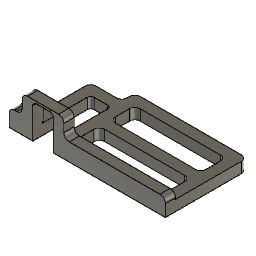
model (Autodesk Fusion 360 design; units mm, degrees)
Autodesk Fusion 360 part; units mm, degrees
note: some values were not read from the file. Set by a fixed rule: which sketch regions a step uses.
sketch "Sketch2" plane through (0, 0, 0) normal (0, 0, 1) x (1, 0, 0) in component "jig"
  line L0 (0, 0) -> (0, 66.75)
  line L1 (0, 66.75) -> (146.025, 66.75)
  line L2 (146.025, 66.75) -> (146.025, 0)
  line L3 (146.025, 0) -> (0, 0)
  line L4 (22.25, 0) -> (41.25, 0)
  line L5 (41.25, 0) -> (41.25, 44.5)
  line L6 (41.25, 44.5) -> (22.25, 44.5)
  line L7 (22.25, 44.5) -> (22.25, 0)
  line L8 (0, 0) -> (22.25, 0)
  line L9 (22.25, 0) -> (22.25, -9.5)
  line L10 (22.25, -9.5) -> (0, -9.5)
  line L11 (0, -9.5) -> (0, 0)
  line L12 (146.025, 0) -> (41.25, 0)
  line L13 (41.25, 0) -> (41.25, -9.5)
  line L14 (41.25, -9.5) -> (146.025, -9.5)
  line L15 (146.025, -9.5) -> (146.025, 0)
  line L16 (22.25, 44.5) -> (0, 44.5) construction
  line L17 (41.25, 44.5) -> (146.025, 44.5) construction
  dimension "d27" = 104.775
  dimension "d29" = 9.5
  dimension "d58" = 19
  dimension "d59" = 22.25
  dimension "d60" = 44.5
  dimension "d64" = 22.25
  constraint coincident L0.start L3.end
  constraint vertical L0
  constraint perpendicular L0 L1
  constraint perpendicular L1 L2
  constraint perpendicular L0 L3
  constraint horizontal L4
  constraint vertical L5
  constraint horizontal L6
  constraint vertical L7
  constraint coincident L3 L4.start
  constraint horizontal L8
  constraint vertical L9
  constraint horizontal L10
  constraint vertical L11
  constraint horizontal L12
  constraint vertical L13
  constraint horizontal L14
  constraint vertical L15
  constraint collinear L10 L14
  constraint collinear L7 L9
  constraint collinear L5 L13
  constraint perpendicular L0 L16
  constraint coincident L0 L16.end
  constraint coincident L2 L17.end
  constraint perpendicular L2 L17
  measures "d27" distance of L2 L5
  measures "d29" distance of L0.start L10.end
  measures "d58" distance of L5.end L6.end
  measures "d59" distance of L1 L6
  measures "d60" distance of L3 L6
  measures "d64" distance of L9.end L10.end
extrude "Extrude1" add sketch "Sketch2" along normal blind 10 contours L0 L1 L2 L3 L5 L6 L7 L8 L12 in component "jig"
extrude "Extrude2" add sketch "Sketch2" along normal blind 33.75 contours L3 L8 L9 L10 L11 | L3 L12 L13 L14 L15 in component "jig"
sketch "Sketch3" plane through (0, 0, 0) normal (-1, 0, 0) x (0, -1, 0) in component "jig"
  line L0 (-66.75, 0) -> (9.5, 0)
  line L1 (9.5, 0) -> (9.5, 33.75)
  line L2 (9.5, 33.75) -> (0, 33.75)
  line L3 (-160, 13) -> (-160.4879, 12.5121)
  line L4 (-160.2757, 12) -> (-160, 12)
  line L5 (-160, 13) -> (-160, 12)
  arc A0 (-160.4879, 12.5121) -> (-160.2757, 12) centre (-160.2757, 12.3) ccw
  line L6 (0, 10) -> (0.2757, 10)
  line L7 (0.4879, 10.5121) -> (0, 11)
  line L8 (0, 10) -> (0, 11)
  arc A1 (0.2757, 10) -> (0.4879, 10.5121) centre (0.2757, 10.3) ccw
  line L9 (-66.75, 10) -> (-66.75, 0)
  line L10 (0, 33.75) -> (0, 10)
  line L11 (0, 10) -> (-66.75, 10)
  dimension "d34" = 1
  dimension "d35" = 0.3
  dimension "d36" = 45
  dimension "d37" = 1
  dimension "d38" = 45
  dimension "d39" = 0.3
  constraint tangent L3 A0
  constraint tangent L4 A0
  constraint tangent L6 A1
  constraint tangent L7 A1
  constraint coincident L6.start L8.start
  measures "d34" distance of L3.start L4.end
  measures "d35" radius of A0
  measures "d36" angle of L3 L5
  measures "d37" distance of L6.start L7.end
  measures "d38" angle of L7 L8
  measures "d39" radius of A1
  measures "d86" radius of A0.centre
extrude "Extrude3" cut sketch "Sketch3" against normal up to surface (146.025 mm away) contours L6 L7 L8 A1 L10 | L3 L4 L5 A0 in component "jig"
fillet "Fillet2" radius 3.175 2 edges at (22.25, 44.5, 5) (41.25, 44.5, 5) in component "jig"
sketch "Sketch2 (2)" plane through (0, -9.5, 0) normal (0, -1, 0) x (1, 0, 0) in component "jig"
  line L0 (0, 0) -> (22.25, 0)
  line L1 (22.25, 0) -> (22.25, 33.75)
  line L2 (22.25, 33.75) -> (0, 33.75)
  line L3 (0, 33.75) -> (0, 0)
  line L4 (22.25, 33.75) -> (41.25, 33.75)
  line L5 (41.25, 0) -> (41.25, 33.75)
  line L6 (41.25, 33.75) -> (41.25, 29.75)
  line L7 (22.25, 33.75) -> (22.25, 29.75)
  line L8 (22.25, 29.75) -> (24.6335, 31.75)
  line L9 (24.6335, 31.75) -> (38.8665, 31.75)
  line L10 (38.8665, 31.75) -> (41.25, 29.75)
  line L11 (22.25, 29.75) -> (41.25, 29.75) construction
  point P0 (41.25, 33.75)
  dimension "d65" = 50
  dimension "d66" = 50
  dimension "d67" = 4
  dimension "d68" = 2
  constraint coincident L1.end L2.start
  constraint coincident P0 L4.end
  constraint coincident L5 L6.end
  constraint perpendicular L4 L6
  constraint coincident L1 L7.end
  constraint perpendicular L2 L7
  constraint perpendicular L1 L9
  constraint horizontal L11
  measures "d65" angle of L7 L8
  measures "d66" angle of L6 L10
  measures "d67" distance of L1.end L7.end
  measures "d68" distance of L4 L9
extrude "Extrude5" add sketch "Sketch2 (2)" against normal up to surface (9.5 mm away) contours L1 L4 L5 L6 L7 L8 L9 L10 in component "jig"
sketch "Sketch3 (2)" plane through (0, 0, 10) normal (0, 0, 1) x (-1, 0, 0) in component "jig"
  line L0 (-25.425, -44.5) -> (-38.075, -44.5)
  arc A0 (-41.25, -41.325) -> (-38.075, -44.5) centre (-38.075, -41.325) ccw
  line L1 (-41.25, -41.325) -> (-41.25, 0.2757)
  line L2 (-41.25, 0.2757) -> (-146.025, 0.2757)
  line L3 (-146.025, 0.2757) -> (-146.025, -66.75)
  line L4 (-146.025, -66.75) -> (0, -66.75)
  line L5 (0, -66.75) -> (0, 0.2757)
  line L6 (0, 0.2757) -> (-22.25, 0.2757)
  line L7 (-22.25, 0.2757) -> (-22.25, -41.325)
  arc A1 (-25.425, -44.5) -> (-22.25, -41.325) centre (-25.425, -41.325) ccw
  line L8 (-56.25, -56.75) -> (-131.025, -56.75)
  line L9 (-136.025, -51.75) -> (-136.025, -38.625)
  line L10 (-131.025, -33.625) -> (-56.25, -33.625)
  line L11 (-51.25, -38.625) -> (-51.25, -51.75)
  line L12 (-146.025, 0) -> (0, 0)
  arc A2 (-56.25, -56.75) -> (-51.25, -51.75) centre (-56.25, -51.75) ccw
  arc A3 (-136.025, -51.75) -> (-131.025, -56.75) centre (-131.025, -51.75) ccw
  arc A4 (-131.025, -33.625) -> (-136.025, -38.625) centre (-131.025, -38.625) ccw
  arc A5 (-51.25, -38.625) -> (-56.25, -33.625) centre (-56.25, -38.625) ccw
  line L13 (-56.25, -0.5) -> (-131.025, -0.5)
  line L14 (-136.025, -5.5) -> (-136.025, -18.625)
  line L15 (-131.025, -23.625) -> (-56.25, -23.625)
  line L16 (-51.25, -18.625) -> (-51.25, -5.5)
  line L17 (0, 9.5) -> (-146.025, 9.5)
  line L18 (-93.6375, -56.75) -> (-93.6375, -33.625) construction
  line L19 (-93.6375, -23.625) -> (-93.6375, -0.5) construction
  arc A6 (-56.25, -23.625) -> (-51.25, -18.625) centre (-56.25, -18.625) ccw
  arc A7 (-51.25, -5.5) -> (-56.25, -0.5) centre (-56.25, -5.5) ccw
  arc A8 (-131.025, -0.5) -> (-136.025, -5.5) centre (-131.025, -5.5) ccw
  arc A9 (-136.025, -18.625) -> (-131.025, -23.625) centre (-131.025, -18.625) ccw
  dimension "d71" = 10
  dimension "d72" = 10
  dimension "d74" = 10
  dimension "d75" = 5
  dimension "d89" = 10
  dimension "d90" = 10
  dimension "d91" = 5
  constraint horizontal L8
  constraint vertical L9
  constraint horizontal L10
  constraint vertical L11
  constraint tangent L8 A2
  constraint tangent L11 A2
  constraint tangent L8 A3
  constraint tangent L9 A3
  constraint equal A2 A3
  constraint tangent L9 A4
  constraint tangent L10 A4
  constraint equal A2 A4
  constraint tangent L10 A5
  constraint tangent L11 A5
  constraint equal A2 A5
  constraint horizontal L13
  constraint vertical L14
  constraint horizontal L15
  constraint vertical L16
  constraint midpoint L8 L18.start
  constraint midpoint L10 L18.end
  constraint equal L18 L19
  constraint coincident L15 L19.start
  constraint tangent L15 A6
  constraint tangent L16 A6
  constraint coincident L13 L19.end
  constraint tangent L13 A7
  constraint tangent L16 A7
  constraint equal A6 A7
  constraint tangent L13 A8
  constraint tangent L14 A8
  constraint equal A6 A8
  constraint tangent L14 A9
  constraint tangent L15 A9
  constraint equal A6 A9
  constraint collinear L11 L16
  constraint collinear L9 L14
  measures "d71" distance of L1 L11
  measures "d72" distance of L4 L8
  measures "d74" distance of L3 L9
  measures "d75" radius of A2
  measures "d89" distance of L10 L15
  measures "d90" distance of L13 L17
  measures "d91" radius of A6
extrude "Extrude6" cut sketch "Sketch3 (2)" against normal up to surface (10 mm away) contours L8 L9 L10 L11 A2 A3 A4 A5 | L13 L14 L15 L16 A6 A7 A8 A9 in component "jig"
sketch "Sketch10" plane through (0, 0, 0) normal (0, 1, 0) x (-1, 0, 0) in component "jig"
  line L0 (-146.025, 11) -> (-41.25, 11)
  line L1 (-41.25, 11) -> (-41.25, 29.75)
  line L2 (-41.25, 29.75) -> (-38.8665, 31.75)
  line L3 (-38.8665, 31.75) -> (-24.6335, 31.75)
  line L4 (-24.6335, 31.75) -> (-22.25, 29.75)
  line L5 (-22.25, 29.75) -> (-22.25, 11)
  line L6 (-22.25, 11) -> (0, 11)
  line L7 (0, 11) -> (0, 33.75)
  line L8 (0, 33.75) -> (-146.025, 33.75)
  line L9 (-146.025, 33.75) -> (-146.025, 11)
  line L10 (-146.025, 49.75) -> (-53.25, 49.75)
  line L11 (-51.25, 28.75) -> (-51.25, 21.3333)
  line L12 (-56.25, 16.3333) -> (-146.025, 16.3333)
  line L13 (-146.025, 16.3333) -> (-146.025, 49.75)
  line L14 (-146.025, 10) -> (0, 10)
  line L15 (0, 49.75) -> (-10.25, 49.75)
  line L16 (-12.25, 28.75) -> (-12.25, 21.3333)
  line L17 (-7.25, 16.3333) -> (0, 16.3333)
  line L18 (0, 16.3333) -> (0, 49.75)
  line L19 (-53.25, 49.75) -> (-10.25, 49.75)
  line L20 (-17.25, 33.75) -> (-46.25, 33.75)
  arc A0 (-56.25, 16.3333) -> (-51.25, 21.3333) centre (-56.25, 21.3333) ccw
  arc A1 (-46.25, 33.75) -> (-51.25, 28.75) centre (-46.25, 28.75) ccw
  arc A2 (-12.25, 28.75) -> (-17.25, 33.75) centre (-17.25, 28.75) ccw
  arc A3 (-12.25, 21.3333) -> (-7.25, 16.3333) centre (-7.25, 21.3333) ccw
  dimension "d81" = 10
  dimension "d82" = 6.3333
  dimension "d83" = 6.3333
  dimension "d84" = 10
  dimension "d85" = 16
  dimension "d86" = 5
  constraint horizontal L10
  constraint vertical L11
  constraint horizontal L12
  constraint vertical L13
  constraint horizontal L15
  constraint vertical L16
  constraint horizontal L17
  constraint vertical L18
  constraint collinear L10 L15
  constraint collinear L9 L13
  constraint horizontal L19
  constraint horizontal L20
  constraint coincident L15.end L19.end
  constraint collinear L7 L18
  constraint tangent L11 A0
  constraint tangent L12 A0
  constraint tangent L20 A1
  constraint tangent L11 A1
  constraint equal A0 A1
  constraint tangent L20 A2
  constraint tangent L16 A2
  constraint equal A0 A2
  constraint tangent L16 A3
  constraint tangent L17 A3
  constraint equal A0 A3
  constraint collinear L8 L20
  measures "d81" distance of L1 L11
  measures "d82" distance of L12 L14
  measures "d83" distance of L14 L17
  measures "d84" distance of L5 L16
  measures "d85" distance of L8 L10
  measures "d86" radius of A0
extrude "Extrude7" cut sketch "Sketch10" against normal up to surface (9.5 mm away) contours L8 L9 L11 L12 L13 A0 A1 | L7 L8 L16 L17 L18 A2 A3 in component "jig"
fillet "Fillet3" radius 5 4 edges at (0, -4.75, 16.3333) (0, 66.75, 5) (146.025, -4.75, 16.3333) (146.025, 66.75, 5) in component "jig"
sketch "Sketch11" plane through (0, 0, 10) normal (0, 0, 1) x (-1, 0, 0) in component "jig"
  arc A0 (-146.025, -61.75) -> (-141.025, -66.75) centre (-141.025, -61.75) ccw
  line L0 (-141.025, -66.75) -> (-5, -66.75)
  arc A1 (-5, -66.75) -> (0, -61.75) centre (-5, -61.75) ccw
  line L1 (0, -61.75) -> (0, 0.2757)
  line L2 (0, 0.2757) -> (-22.25, 0.2757)
  line L3 (-22.25, 0.2757) -> (-22.25, -41.325)
  arc A2 (-25.425, -44.5) -> (-22.25, -41.325) centre (-25.425, -41.325) ccw
  line L4 (-25.425, -44.5) -> (-38.075, -44.5)
  arc A3 (-41.25, -41.325) -> (-38.075, -44.5) centre (-38.075, -41.325) ccw
  line L5 (-41.25, -41.325) -> (-41.25, 0.2757)
  line L6 (-41.25, 0.2757) -> (-146.025, 0.2757)
  line L7 (-146.025, 0.2757) -> (-146.025, -61.75)
  line L8 (-136.025, -51.75) -> (-136.025, -38.625)
  arc A4 (-131.025, -33.625) -> (-136.025, -38.625) centre (-131.025, -38.625) ccw
  line L9 (-131.025, -33.625) -> (-56.25, -33.625)
  arc A5 (-51.25, -38.625) -> (-56.25, -33.625) centre (-56.25, -38.625) ccw
  line L10 (-51.25, -38.625) -> (-51.25, -51.75)
  arc A6 (-56.25, -56.75) -> (-51.25, -51.75) centre (-56.25, -51.75) ccw
  line L11 (-56.25, -56.75) -> (-131.025, -56.75)
  arc A7 (-136.025, -51.75) -> (-131.025, -56.75) centre (-131.025, -51.75) ccw
  line L12 (-131.025, -0.5) -> (-56.25, -0.5)
  arc A8 (-51.25, -5.5) -> (-56.25, -0.5) centre (-56.25, -5.5) ccw
  line L13 (-51.25, -5.5) -> (-51.25, -18.625)
  arc A9 (-56.25, -23.625) -> (-51.25, -18.625) centre (-56.25, -18.625) ccw
  line L14 (-56.25, -23.625) -> (-131.025, -23.625)
  arc A10 (-136.025, -18.625) -> (-131.025, -23.625) centre (-131.025, -18.625) ccw
  line L15 (-136.025, -18.625) -> (-136.025, -5.5)
  arc A11 (-131.025, -0.5) -> (-136.025, -5.5) centre (-131.025, -5.5) ccw
  line L16 (0, -10) -> (-12.25, -10)
  line L17 (-12.25, -10) -> (-12.25, -54.5)
  line L18 (-12.25, -54.5) -> (-41.25, -54.5)
  line L19 (-41.25, -54.5) -> (-41.25, -66.75)
  line L20 (0, -10) -> (0, -66.75)
  line L21 (0, -66.75) -> (-41.25, -66.75)
  line L22 (-46.25, 0) -> (-17.25, 0)
  dimension "d94" = 10
  dimension "d95" = 10
  dimension "d96" = 10
  constraint coincident L1 L16.start
  constraint perpendicular L1 L16
  constraint perpendicular L16 L17
  constraint perpendicular L17 L18
  constraint coincident L0 L19.end
  constraint perpendicular L0 L19
  constraint perpendicular L16 L20
  constraint perpendicular L19 L21
  constraint collinear L5 L19
  measures "d94" distance of L4 L18
  measures "d95" distance of L3 L17
  measures "d96" distance of L16 L22
extrude "Extrude8" cut sketch "Sketch11" against normal up to surface (10 mm away) contours L0 A1 L1 L16 L17 L18 L19 L20 L21 in component "jig"
fillet "Fillet4" radius 5 5 edges at (41.25, 66.75, 5) (41.25, 54.5, 5) (12.25, 54.5, 5) (12.25, 10, 5) (0, 10, 5) in component "jig"
fillet "Fillet5" radius 2 4 edges at (22.25, -4.75, 29.75) (24.6335, -4.75, 31.75) (38.8665, -4.75, 31.75) (41.25, -4.75, 29.75) in component "jig"
component "jig" placed x (1, 0, 0) y (0, 1, 0) z (0, 0, 1) at (0, 0, 0)
equation "stockW = 200 mm"
equation "stockH = 89 mm"
equation "stockT = 19 mm"
equation "lipT = stockT / 2"
equation "lipH = lipT * 2 / 3"
equation "jigT = 10 mm"
equation "stock2H = 160 mm"
equation "baseMargin = 3.125 in + 1\""
equation "d27 = baseMargin"
equation "d29 = lipT"
equation "d30 = jigT"
equation "d32 = jigT + stockT * 1.25"
equation "d58 = stockT"
equation "d59 = d60 / 2"
equation "d60 = stockH / 2"
equation "jigR = 0.125 in"
equation "d63 = jigR"
equation "d64 = d59"
equation "d66 = d65"
equation "d71 = cutoutOffset"
equation "d72 = d71"
equation "d74 = d71"
equation "d75 = cutoutRadius"
equation "cutoutOffset = 10 mm"
equation "cutoutRadius = 5 mm"
equation "d81 = cutoutOffset"
equation "d82 = lipH"
equation "d83 = lipH"
equation "d84 = cutoutOffset"
equation "d86 = cutoutRadius"
equation "d89 = cutoutOffset"
equation "d90 = cutoutOffset"
equation "d91 = d75"
equation "d93 = cutoutRadius"
equation "d94 = cutoutOffset"
equation "d95 = cutoutOffset"
equation "d96 = cutoutOffset"
equation "d100 = cutoutRadius"
